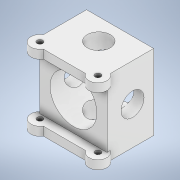
# Autodesk Inventor part: testPrintBracketV2
Saved by Autodesk Inventor 2022 (Build 260153000, 153)
## iProperties
Created: 2022-02-05
Part Number: testPrintBracketV2
Material: Generic
Document SubType Name: Modeling
Designer: ultra
Density: 1 g/cm^3
Appearance: Smooth - White
Author: ultra
Autodesk Inventor part; units mm, degrees
ref_plane "YZ Plane" through (0, 0, 0) normal (1, 0, 0) x (0, 1, 0)
ref_plane "XZ Plane" through (0, 0, 0) normal (0, 1, 0) x (-1, 0, 0)
ref_plane "XY Plane" through (0, 0, 0) normal (0, 0, 1) x (1, 0, 0)
sketch "Sketch2" plane through (0, 0, 0) normal (1, 0, 0) x (0, 1, 0)
  circle A0 centre (0, 0) radius 12.881
  line L0 (-16, -18.5) -> (16, -18.5)
  line L1 (16, -18.5) -> (16, 18.5)
  line L2 (16, 18.5) -> (-16, 18.5)
  line L3 (-16, 18.5) -> (-16, -18.5)
  line L4 (-16, -18.5) -> (16, 18.5) construction
  line L5 (16, -18.5) -> (-16, 18.5) construction
  dimension "d9" = 25.762
  dimension "d10" = 32
  dimension "d11" = 37
  constraints: 12 end point, 2 midpoint, 2 parallel, 1 centre point, 1 coincident, 1 horizontal, 1 perpendicular
  measures "d9" diameter of A0
  measures "d10" distance of L2.end L1.end
  measures "d11" distance of L1.end L0.end
extrude "Extrusion2" add sketch "Sketch2" along normal blind 76.2
sketch "Sketch3" plane through (0, -16, -18.5) normal (0, 0, -1) x (-1, 0, 0)
  line L0 (0, 0) -> (0, 32) projected
  circle A0 centre (18.5, 16) radius 12.881
  line L1 (0, 32) -> (0, 0)
  line L2 (0, 0) -> (37, 0)
  line L3 (37, 0) -> (37, 32)
  line L4 (37, 32) -> (0, 32)
  line L5 (0, 32) -> (37, 0) construction
  line L6 (0, 0) -> (37, 32) construction
  point P0 (0, 16)
  dimension "d14" = 25.762
  dimension "d15" = 32
  dimension "d16" = 37
  constraints: 12 end point, 2 midpoint, 2 parallel, 1 centre point, 1 coincident, 1 perpendicular
  measures "d14" diameter of A0
  measures "d15" distance of L3.end L2.end
  measures "d16" distance of L2.end L1.end
extrude "Extrusion3" add sketch "Sketch3" against normal blind 113.2
sketch "Sketch4" plane through (76.2, -16, -18.5) normal (0, 0, -1) x (-1, 0, 0)
  circle A0 centre (94.7, 16) radius 12.881 projected
  point P0 (76.2, 16)
extrude "Extrusion4" add sketch "Sketch4" against normal blind 37
sketch "Sketch5" plane through (76.2, 16, 18.5) normal (0, 1, 0) x (1, 0, 0)
  line L0 (-113.2, 37) -> (0, 37) projected
  line L1 (-113.2, 37) -> (-113.2, -76.2) projected
  line L2 (-113.2, 37) -> (-100.1185, 50.0815)
  line L3 (-113.2, 37) -> (-94.7, 37) construction
  line L4 (-113.2, 37) -> (-126.2815, 23.9185)
  line L5 (-113.2, 37) -> (-94.7, 37) construction
  line L6 (-100.1185, 50.0815) -> (-154.0001, 103.963)
  line L7 (-126.2815, 23.9185) -> (-180.163, 77.8001)
  line L8 (-126.2815, 23.9185) -> (-50.0815, 23.9185) construction
  line L9 (-154.0001, 103.963) -> (-180.163, 77.8001)
  line L10 (-100.1185, 50.0815) -> (-87.037, 37)
  line L11 (-126.2815, 23.9185) -> (-113.2, 10.837)
  point P0 (-76.2, 18.5)
  dimension "d21" = 18.5
  dimension "d22" = 45
  dimension "d23" = 18.5
  dimension "d24" = 135
  dimension "d25" = 76.2
  dimension "d26" = 76.2
  dimension "d27" = 135
  constraints: 20 end point, 3 equal length, 3 horizontal, 2 point on line
  measures "d21" distance of L0.start L2.end
  measures "d22" angle of L3 L2
  measures "d23" distance of L0.start L4.end
  measures "d24" angle of L4 L5
  measures "d25" distance of L2.end L6.end
  measures "d26" distance of L4.end L7.end
  measures "d27" angle of L8 L7
extrude "Extrusion5" add sketch "Sketch5" against normal blind 32
sketch "Sketch7" plane through (-77.8001, -16, -85.463) normal (-0.7071068, 0, -0.7071068) x (-0.7071068, 0, 0.7071068)
  line L0 (36.4256, 0.4968) -> (36.4256, 31.5032)
  line L1 (36.4256, 31.5032) -> (0.5744, 31.5032)
  line L2 (0.5744, 31.5032) -> (0.5744, 0.4968)
  line L3 (0.5744, 0.4968) -> (36.4256, 0.4968)
  circle A0 centre (18.5, 16) radius 12.881
  point P0 (5.4185, 16)
  point P1 (36.4256, 16)
  dimension "d131" = 25.762
  constraints: 8 end point, 1 centre point
  measures "d131" diameter of A0
extrude "Extrusion6" cut sketch "Sketch7" against normal blind 101.6 contours A0
sketch "Sketch8" plane through (76.2, 16, 18.5) normal (0, 1, 0) x (1, 0, 0)
  line L0 (-76.2, 0) -> (0, 0) projected
  line L1 (-87.037, 37) -> (0, 37) projected
  line L2 (-87.037, 37) -> (-154.0001, 103.963) projected
  line L3 (-180.163, 77.8001) -> (-113.2, 10.837) projected
  line L4 (-113.2, 10.837) -> (-113.2, -76.2) projected
  line L5 (-76.2, 0) -> (-76.2, -76.2) projected
  line L6 (0, 37) -> (5, 37)
  line L7 (5, 37) -> (5, 0)
  line L8 (5, 0) -> (0, 0)
  line L9 (0, 0) -> (0, 37)
  line L10 (-113.2, -76.2) -> (-76.2, -76.2)
  line L11 (-76.2, -76.2) -> (-76.2, -81.2)
  line L12 (-76.2, -81.2) -> (-113.2, -81.2)
  line L13 (-113.2, -81.2) -> (-113.2, -76.2)
  line L14 (-180.163, 77.8001) -> (-183.6985, 81.3356)
  line L15 (-183.6985, 81.3356) -> (-157.5356, 107.4985)
  line L16 (-157.5356, 107.4985) -> (-154.0001, 103.963)
  point P0 (-76.2, 18.5)
  dimension "d32" = 5
  dimension "d33" = 5
  dimension "d34" = 5
  dimension "d35" = 90
  constraints: 22 end point, 4 parallel, 3 perpendicular, 2 horizontal
  measures "d32" distance of L7.end L8.end
  measures "d33" distance of L10.end L11.end
  measures "d34" distance of L3.start L14.end
  measures "d35" angle of L14 L15
extrude "Extrusion7" add sketch "Sketch8" along normal blind 4.7752
sketch "Sketch9" plane through (76.2, -16, -18.5) normal (0, -1, 0) x (1, 0, 0)
  line L0 (-87.037, 0) -> (0, 0) projected
  line L1 (-76.2, 37) -> (0, 37) projected
  line L2 (-76.2, 37) -> (-76.2, 113.2) projected
  line L3 (-113.2, 26.163) -> (-113.2, 113.2) projected
  line L4 (-113.2, 26.163) -> (-180.163, -40.8001) projected
  line L5 (-154.0001, -66.963) -> (-87.037, 0) projected
  line L6 (-76.2, 118.2) -> (-76.2, 37) projected
  line L7 (-113.2, 113.2) -> (-76.2, 113.2)
  line L8 (-76.2, 113.2) -> (-76.2, 118.2)
  line L9 (-76.2, 118.2) -> (-113.2, 118.2)
  line L10 (-113.2, 118.2) -> (-113.2, 113.2)
  line L11 (-76.2, 37) -> (5, 37) projected
  line L12 (0, 0) -> (5, 0)
  line L13 (5, 0) -> (5, 37)
  line L14 (5, 37) -> (0, 37)
  line L15 (0, 37) -> (0, 0)
  line L16 (-183.6985, -44.3356) -> (-113.2, 26.163) projected
  line L17 (-180.163, -40.8001) -> (-183.6985, -44.3356)
  line L18 (-183.6985, -44.3356) -> (-157.5356, -70.4985)
  line L19 (-157.5356, -70.4985) -> (-154.0001, -66.963)
  point P0 (-76.2, 18.5)
  constraints: 22 end point, 4 parallel, 4 perpendicular, 2 horizontal, 1 collinear
extrude "Extrusion8" add sketch "Sketch9" along normal blind 4.7752
sketch "Sketch10" plane through (76.2, 20.7752, 18.5) normal (0, 1, 0) x (1, 0, 0)
  circle A0 centre (2.5, 34.5) radius 1.5875
  circle A1 centre (2.5, 2.5) radius 1.5875
  line L0 (0, 37) -> (0, 0)
  line L1 (0, 0) -> (5, 0)
  line L2 (5, 37) -> (5, 0)
  line L3 (0, 37) -> (5, 37)
  point P0 (-76.2, 18.5)
  point P1 (0, 18.5)
  constraints: 8 end point, 2 centre point
extrude "Extrusion9" cut sketch "Sketch10" against normal blind 279.4 contours A0 | A1
sketch "Sketch11" plane through (76.2, 20.7752, 18.5) normal (0, 1, 0) x (1, 0, 0)
  circle A0 centre (-78.7, -78.7) radius 1.5875
  circle A1 centre (-110.7, -78.7) radius 1.5875
  line L0 (-76.2, -76.2) -> (-113.2, -76.2)
  line L1 (-113.2, -76.2) -> (-113.2, -81.2)
  line L2 (-76.2, -81.2) -> (-113.2, -81.2)
  line L3 (-76.2, -76.2) -> (-76.2, -81.2)
  circle A2 centre (-157.5356, 103.963) radius 1.5875
  circle A3 centre (-180.163, 81.3356) radius 1.5875
  line L4 (-157.5356, 107.4985) -> (-183.6985, 81.3356)
  line L5 (-183.6985, 81.3356) -> (-180.163, 77.8001)
  line L6 (-154.0001, 103.963) -> (-180.163, 77.8001)
  line L7 (-157.5356, 107.4985) -> (-154.0001, 103.963)
  point P0 (-76.2, 18.5)
  point P1 (-94.7, -76.2)
  point P2 (-170.6171, 94.4171)
  constraints: 16 end point, 4 centre point
extrude "Extrusion10" cut sketch "Sketch11" against normal blind 279.4 contours A0 | A1 | A2 | A3
fillet "Fillet1" radius 3.175 3 edges at (-10.837, 0, -18.5) (0, 0, 18.5) (-37, 0, 7.663)
sketch "Sketch13" plane through (76.2, 20.7752, 18.5) normal (0, 1, 0) x (1, 0, 0)
  line L0 (-157.5356, 107.4985) -> (-183.6985, 81.3356) projected
  line L1 (-113.2, -81.2) -> (-76.2, -81.2) projected
  line L2 (5, 0) -> (5, 37) projected
  line L3 (5, 37) -> (5, 0) projected
  line L4 (5, 18.5) -> (-120.863, 18.5)
  line L5 (-114.1299, 11.767) -> (-183.6985, 81.3356) projected
  line L6 (-76.2, -81.2) -> (-113.2, -81.2) projected
  line L7 (-94.7, -81.2) -> (-95.2395, 19.0395)
  line L8 (-104.3477, 9.9312) -> (-86.1312, 28.1477) projected
  line L9 (-95.2395, 19.0395) -> (-170.6171, 94.4171)
  line L10 (-183.6985, 81.3356) -> (-157.5356, 107.4985) projected
  circle A0 centre (-14.05, 18.5) radius 6.35
  circle A1 centre (-39.45, 18.5) radius 6.35
  circle A2 centre (-64.85, 18.5) radius 6.35
  circle A3 centre (-90.25, 18.5) radius 6.35
  circle A4 centre (-94.8025, -62.15) radius 6.35
  circle A5 centre (-94.9392, -36.7504) radius 6.35
  circle A6 centre (-95.0759, -11.3507) radius 6.35
  circle A7 centre (-95.2126, 14.0489) radius 6.35
  circle A8 centre (-157.1467, 80.9467) radius 6.35
  circle A9 centre (-139.1862, 62.9862) radius 6.35
  circle A10 centre (-121.2257, 45.0257) radius 6.35
  circle A11 centre (-103.2651, 27.0651) radius 6.35
  point P0 (-76.2, 18.5)
  point P1 (-95.1101, -5.0008)
  point P2 (-95.0418, -17.7006)
  point P3 (-94.9734, -30.4005)
  point P4 (-94.9051, -43.1003)
  dimension "d60" = 12.7
  dimension "d61" = 19.05
  dimension "d64" = 25.4
  dimension "d69" = 12.7
  dimension "d70" = 19.05
  dimension "d73" = 25.4
  dimension "d78" = 12.7
  dimension "d79" = 19.05
  dimension "d82" = 25.4
  constraints: 12 centre point, 6 end point, 4 midpoint, 4 point on line, 2 horizontal, 20 other
  measures "d60" diameter of A0
  measures "d61" distance from line of L2 A0.centre
  measures "d64" distance of A0.centre A1.centre
  measures "d69" diameter of A4
  measures "d70" distance from line of L1 A4.centre
  measures "d73" distance of A4.centre A5.centre
  measures "d78" diameter of A8
  measures "d79" distance from line of L0 A8.centre
  measures "d82" distance of A8.centre A9.centre
extrude "Extrusion12" cut sketch "Sketch13" against normal blind 127 contours A8 L9 | L9 A8 | A9 L9 | L9 A9 | A11 L9 | L9 A11 | A10 L9 | L9 A10 | A0 L4 | L4 A0 | A1 L4 | L4 A1 | A2 L4 | L4 A2 | A4 L7 | L7 A4 | A5 L7 | L7 A5 | A6 L7 | L7 A6
sketch "Sketch14" plane through (81.2, 16, -18.5) normal (0, 0, -1) x (-1, 0, 0)
  line L0 (0, 4.7752) -> (90.7219, 4.7752) projected
  line L1 (0, 0) -> (0, 4.7752) projected
  circle A0 centre (19.05, -16) radius 6.35
  circle A1 centre (44.45, -16) radius 6.35
  circle A2 centre (69.85, -16) radius 6.35
  point P0 (81.2, -16)
  dimension "d89" = 12.7
  dimension "d91" = 19.05
  dimension "d94" = 25.4
  constraints: 3 centre point, 1 horizontal, 4 other
  measures "d89" diameter of A0
  measures "d91" distance from line of A0.centre L1
  measures "d94" distance of A0.centre A1.centre
extrude "Extrusion13" cut sketch "Sketch14" against normal blind 50.8
sketch "Sketch15" plane through (-37, 16, 94.7) normal (-1, 0, 0) x (0, 0, 1)
  line L0 (5, 0) -> (5, 4.7752) projected
  line L1 (-85.7219, 4.7752) -> (5, 4.7752) projected
  circle A0 centre (-14.05, -16) radius 6.35
  circle A1 centre (-39.45, -16) radius 6.35
  circle A2 centre (-64.85, -16) radius 6.35
  point P0 (-94.7, -16)
  dimension "d101" = 12.7
  dimension "d102" = 19.05
  dimension "d105" = 25.4
  constraints: 3 centre point, 1 horizontal, 4 other
  measures "d101" diameter of A0
  measures "d102" distance from line of L0 A0.centre
  measures "d105" distance of A0.centre A1.centre
extrude "Extrusion14" cut sketch "Sketch15" against normal blind 50.8
sketch "Sketch16" plane through (-107.4985, 16, -62.8356) normal (-0.7071068, 0, 0.7071068) x (0.7071068, 0, 0.7071068)
  line L0 (0, 4.7752) -> (98.3849, 4.7752) projected
  line L1 (0, 0) -> (0, 4.7752) projected
  circle A0 centre (19.05, -16) radius 6.35
  circle A1 centre (44.45, -16) radius 6.35
  circle A2 centre (69.85, -16) radius 6.35
  point P0 (120.4444, -16)
  dimension "d112" = 12.7
  dimension "d113" = 19.05
  dimension "d116" = 25.4
  constraints: 3 centre point, 1 horizontal, 4 other
  measures "d112" diameter of A0
  measures "d113" distance from line of L1 A0.centre
  measures "d116" distance of A0.centre A1.centre
extrude "Extrusion15" cut sketch "Sketch16" against normal blind 101.6
sketch "Sketch19" plane through (76.2, 20.7752, 18.5) normal (0, 1, 0) x (1, 0, 0)
  circle A0 centre (-157.5356, 103.963) radius 1.5875 projected
  circle A1 centre (-78.7, -78.7) radius 1.5875 projected
  circle A2 centre (-180.163, 81.3356) radius 1.5875 projected
  circle A3 centre (-110.7, -78.7) radius 1.5875 projected
  circle A4 centre (2.5, 2.5) radius 1.5875 projected
  circle A5 centre (2.5, 34.5) radius 1.5875 projected
  line L0 (-87.967, 37.9299) -> (-157.5356, 107.4985) projected
  line L1 (-157.5356, 107.4985) -> (-183.6985, 81.3356) projected
  line L2 (-183.6985, 81.3356) -> (-114.1299, 11.767) projected
  line L3 (-113.2, 9.5219) -> (-113.2, -81.2) projected
  line L4 (-113.2, -81.2) -> (-76.2, -81.2) projected
  line L5 (-76.2, -81.2) -> (-76.2, -3.175) projected
  line L6 (-73.025, 0) -> (5, 0) projected
  line L7 (5, 0) -> (5, 37) projected
  line L8 (5, 37) -> (-85.7219, 37) projected
  circle A6 centre (2.5, 2.5) radius 5
  circle A7 centre (2.5, 34.5) radius 5
  circle A8 centre (-110.7, -78.7) radius 5
  circle A9 centre (-78.7, -78.7) radius 5
  circle A10 centre (-180.163, 81.3356) radius 5
  circle A11 centre (-157.5356, 103.963) radius 5
  point P0 (-76.2, 18.5)
  point P1 (-76.2, -74.3699)
  point P2 (-83.0301, -81.2)
  point P3 (-113.2, -74.3699)
  point P4 (-106.3699, -81.2)
  point P5 (-178.8689, 86.1652)
  point P6 (-178.8689, 76.506)
  point P7 (-152.706, 102.6689)
  point P8 (-162.3652, 102.6689)
  point P9 (5, 6.8301)
  point P10 (-1.8301, 0)
  point P11 (-1.8301, 37)
  point P12 (5, 30.1699)
  dimension "d132" = 10
  dimension "d133" = 10
  dimension "d134" = 10
  dimension "d135" = 10
  dimension "d136" = 10
  dimension "d137" = 10
  constraints: 6 centre point, 6 coincident
  measures "d132" diameter of A6
  measures "d133" diameter of A7
  measures "d134" diameter of A8
  measures "d135" diameter of A9
  measures "d136" diameter of A10
  measures "d137" diameter of A11
extrude "Extrusion17" add sketch "Sketch19" against normal blind 4.7752 contours L0 L1 A11 | L1 L2 A10 | L3 L4 A8 | L4 L5 A9 | L6 L7 A6 | L7 L8 A7 picked at (-160.8118, 104.679) picked at (-180.881, 84.6119) picked at (-108.8911, -81.5244) picked at (-80.5163, -81.5168) picked at (0.6837, -0.3168) picked at (0.6837, 37.3168)
sketch "Sketch20" plane through (76.2, -20.7752, -18.5) normal (0, -1, 0) x (1, 0, 0)
  circle A0 centre (-157.5356, -66.963) radius 1.5875 projected
  circle A1 centre (-180.163, -44.3356) radius 1.5875 projected
  circle A2 centre (2.5, 34.5) radius 1.5875 projected
  circle A3 centre (2.5, 2.5) radius 1.5875 projected
  line L0 (-157.5356, -70.4985) -> (-87.967, -0.9299) projected
  line L1 (-85.7219, 0) -> (5, 0) projected
  line L2 (5, 0) -> (5, 37) projected
  line L3 (5, 37) -> (-73.025, 37) projected
  line L4 (-76.2, 40.175) -> (-76.2, 118.2) projected
  line L5 (-76.2, 118.2) -> (-113.2, 118.2) projected
  line L6 (-113.2, 118.2) -> (-113.2, 27.4781) projected
  line L7 (-114.1299, 25.233) -> (-183.6985, -44.3356) projected
  line L8 (-183.6985, -44.3356) -> (-157.5356, -70.4985) projected
  circle A4 centre (-157.5356, -66.963) radius 5
  circle A5 centre (-180.163, -44.3356) radius 5
  circle A6 centre (-110.7, 115.7) radius 1.5875 projected
  circle A7 centre (-110.7, 115.7) radius 5
  circle A8 centre (-78.7, 115.7) radius 1.5875 projected
  circle A9 centre (-78.7, 115.7) radius 5
  circle A10 centre (2.5, 34.5) radius 5
  circle A11 centre (2.5, 2.5) radius 5
  point P0 (-76.2, 18.5)
  point P1 (5, 6.8301)
  point P2 (-1.8301, 0)
  point P3 (-1.8301, 37)
  point P4 (5, 30.1699)
  point P5 (-83.0301, 118.2)
  point P6 (-76.2, 111.3699)
  point P7 (-106.3699, 118.2)
  point P8 (-113.2, 111.3699)
  point P9 (-162.3652, -65.6689)
  point P10 (-152.706, -65.6689)
  point P11 (-178.8689, -39.506)
  point P12 (-178.8689, -49.1652)
  constraints: 6 centre point, 6 coincident
extrude "Extrusion18" add sketch "Sketch20" against normal blind 4.7752 contours L0 A4 L8 | L1 L2 A11 | L2 L3 A10 | L4 L5 A9 | L5 L6 A7 | L7 L8 A5 picked at (-160.8118, -67.679) picked at (0.6837, -0.3168) picked at (0.6837, 37.3168) picked at (-80.5163, 118.5168) picked at (-113.5244, 113.8911) picked at (-180.881, -47.6119)
sketch "Sketch21" plane through (76.2, 20.7752, 18.5) normal (0, 1, 0) x (1, 0, 0)
  circle A0 centre (-103.2651, 27.0651) radius 6.35 projected
  circle A1 centre (-14.05, 18.5) radius 6.35 projected
  circle A2 centre (-157.1467, 80.9467) radius 6.35 projected
  circle A3 centre (-95.0759, -11.3507) radius 6.35 projected
  circle A4 centre (-121.2257, 45.0257) radius 6.35 projected
  circle A5 centre (-39.45, 18.5) radius 6.35 projected
  circle A6 centre (-64.85, 18.5) radius 6.35 projected
  circle A7 centre (-139.1862, 62.9862) radius 6.35 projected
  circle A8 centre (-94.9392, -36.7504) radius 6.35 projected
  circle A9 centre (-157.5356, 103.963) radius 1.5875 projected
  circle A10 centre (-180.163, 81.3356) radius 1.5875 projected
  circle A11 centre (2.5, 2.5) radius 1.5875 projected
  circle A12 centre (2.5, 34.5) radius 1.5875 projected
  line L0 (-201.6081, 114.1304) -> (16.4266, 114.1304)
  line L1 (16.4266, 114.1304) -> (16.4266, -50.4697)
  line L2 (16.4266, -50.4697) -> (-201.6081, -50.4697)
  line L3 (-201.6081, -50.4697) -> (-201.6081, 114.1304)
  point P0 (-76.2, 18.5)
  constraints: 8 end point, 2 parallel, 1 horizontal, 1 perpendicular
extrude "Extrusion19" cut sketch "Sketch21" against normal blind 76.2
body "Solid2"
